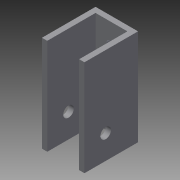
# Autodesk Inventor part: Actuator Bracket
Saved by Autodesk Inventor 2015 (Build 190159000, 159)
## iProperties
Created: 2015-02-16
Part Number: Actuator Bracket
Material: Generic
Document SubType Name: Modeling
Designer: pltwe4
Density: 1 g/cm^3
Appearance: Default
Author: pltwe4
Autodesk Inventor part; units mm, degrees
ref_plane "YZ Plane" through (0, 0, 0) normal (1, 0, 0) x (0, 1, 0)
ref_plane "XZ Plane" through (0, 0, 0) normal (0, 1, 0) x (-1, 0, 0)
ref_plane "XY Plane" through (0, 0, 0) normal (0, 0, 1) x (1, 0, 0)
sketch "Sketch1" plane through (0, 0, 0) normal (0, 1, 0) x (-1, 0, 0)
  line L0 (9.525, 0) -> (9.525, -28.8544)
  line L1 (9.525, -28.8544) -> (-9.525, -28.8544)
  line L2 (-9.525, -28.8544) -> (-9.525, 0)
  line L3 (-9.525, 0) -> (-12.7, 0)
  line L4 (-12.7, 0) -> (-12.7, -32.0294)
  line L5 (-12.7, -32.0294) -> (12.7, -32.0294)
  line L6 (12.7, -32.0294) -> (12.7, 0)
  line L7 (12.7, 0) -> (9.525, 0)
  line L8 (0, -38.4353) -> (0, 6.4059) projected
  line L9 (-17.78, 0) -> (17.78, 0) projected
  point P0 (0, 0)
  dimension "d0" = 3.175
  dimension "d1" = 19.05
  dimension "d2" = 28.8544
  dimension "d3" = 3.175
  constraints: 16 end point, 7 perpendicular, 1 collinear, 1 point on line, 1 vertical, 2 other
  measures "d0" distance between parallel lines of L6 L0
  measures "d1" distance of L0.end L1.end
  measures "d2" distance between parallel lines of L3 L1
  measures "d3" distance between parallel lines of L5 L1
extrude "Extrusion1" add sketch "Sketch1" along normal mid plane 57.404 contours L7 L6 L5 L8 L1 L0 | L8 L5 L4 L3 L2 L1
sketch "Sketch2" plane through (12.7, 28.702, -32.0294) normal (0, 0, -1) x (-1, 0, 0)
  line L0 (25.4, -57.404) -> (25.4, 0) projected
  line L1 (0, 0) -> (25.4, 0) projected
  line L2 (0, -57.404) -> (0, 0) projected
  line L3 (25.4, -57.404) -> (0, -57.404) projected
  line L4 (12.7, -68.8848) -> (12.7, 11.4808) projected
  line L5 (-5.08, -28.702) -> (30.48, -28.702) projected
  circle A0 centre (12.7, -12.7) radius 3.175
  circle A1 centre (12.7, -44.704) radius 3.175
  point P0 (12.7, -28.702)
  dimension "d6" = 6.35
  dimension "d7" = 16.002
  constraints: 2 centre point, 2 point on line, 1 other
  measures "d6" diameter of A0
  measures "d7" distance from line of L5 A0.centre
extrude "Extrusion2" cut sketch "Sketch2" against normal up to next contours A1 L4 | L4 A1 | A0 L4 | L4 A0
sketch "Sketch3" plane through (12.7, -28.702, -32.0294) normal (1, 0, 0) x (0, 0, -1)
  line L0 (0, 0) -> (0, 57.404) projected
  line L1 (-32.0294, 57.404) -> (0, 57.404) projected
  line L2 (-32.0294, 0) -> (-32.0294, 57.404) projected
  line L3 (0, 0) -> (-32.0294, 0) projected
  circle A0 centre (-19.3294, 14.4272) radius 3.175
  point P0 (-32.0294, 28.702)
  dimension "d10" = 6.35
  dimension "d11" = 12.7
  dimension "d12" = 14.4272
  constraints: 1 centre point
  measures "d10" diameter of A0
  measures "d11" distance from line of L2 A0.centre
  measures "d12" distance from line of L3 A0.centre
extrude "Extrusion3" cut sketch "Sketch3" against normal up to surface (25.4 mm away) contours A0
body "Solid1"
